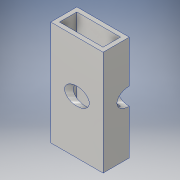
# Autodesk Inventor part: postForAxel
Saved by Autodesk Inventor 2016 SP1 (Build 200210100, 210)
## iProperties
Created: 2016-02-07
Part Number: postForAxel
Material: Aluminum 6061
Document SubType Name: Modeling
Designer: steele
Density: 2.7 g/cm^3
Appearance: Aluminum - Flat
Author: steele
Autodesk Inventor part; units mm, degrees
ref_plane "YZ Plane" through (0, 0, 0) normal (1, 0, 0) x (0, 1, 0)
ref_plane "XZ Plane" through (0, 0, 0) normal (0, 1, 0) x (-1, 0, 0)
sketch "Sketch1" plane through (0, 0, 0) normal (0, 1, 0) x (-1, 0, 0)
  line L0 (19.05, 9.525) -> (-19.05, 9.525)
  line L1 (-19.05, 9.525) -> (-19.05, -9.525)
  line L2 (-19.05, -9.525) -> (19.05, -9.525)
  line L3 (19.05, -9.525) -> (19.05, 9.525)
  line L4 (19.05, 9.525) -> (-19.05, -9.525) construction
  line L5 (-19.05, 9.525) -> (19.05, -9.525) construction
  line L6 (15.875, 6.35) -> (-15.875, 6.35)
  line L7 (-15.875, 6.35) -> (-15.875, -6.35)
  line L8 (-15.875, -6.35) -> (15.875, -6.35)
  line L9 (15.875, -6.35) -> (15.875, 6.35)
  line L10 (15.875, 6.35) -> (-15.875, -6.35) construction
  line L11 (-15.875, 6.35) -> (15.875, -6.35) construction
  point P0 (0, 0)
  dimension "d0" = 19.05
  dimension "d1" = 38.1
  dimension "d2" = 3.175
  dimension "d3" = 3.175
  constraints: 24 end point, 4 midpoint, 4 parallel, 2 horizontal, 2 perpendicular
  measures "d0" distance of L2.end L0.start
  measures "d1" distance of L1.end L2.end
  measures "d2" distance between parallel lines of L0 L6
  measures "d3" distance between parallel lines of L1 L7
extrude "Extrusion1" add sketch "Sketch1" against normal blind 76.2
ref_plane "Work Plane1" through (-19.05, 0, 9.525) normal (-0.7071, 0, 0.7071) x (0, -1, 0)
sketch "Sketch2" plane through (-19.05, 0, 9.525) normal (-0.7071, 0, 0.7071) x (0, -1, 0)
  line L0 (0, 13.4704) -> (76.2, 13.4704) projected
  circle A0 centre (37.211, 13.4704) radius 6.35
  line L1 (0, 0) -> (0, 26.9408) projected
  point P0 (0, 6.7352)
  dimension "d7" = 12.7
  dimension "d10" = 37.211
  constraints: 1 centre point, 1 point on line
  measures "d7" diameter of A0
  measures "d10" distance from line of A0.centre L1
extrude "Extrusion2" cut sketch "Sketch2" against normal through all
equation "\"d4\" = length"
equation "\"length\" = 76.2"
body "Solid1"
